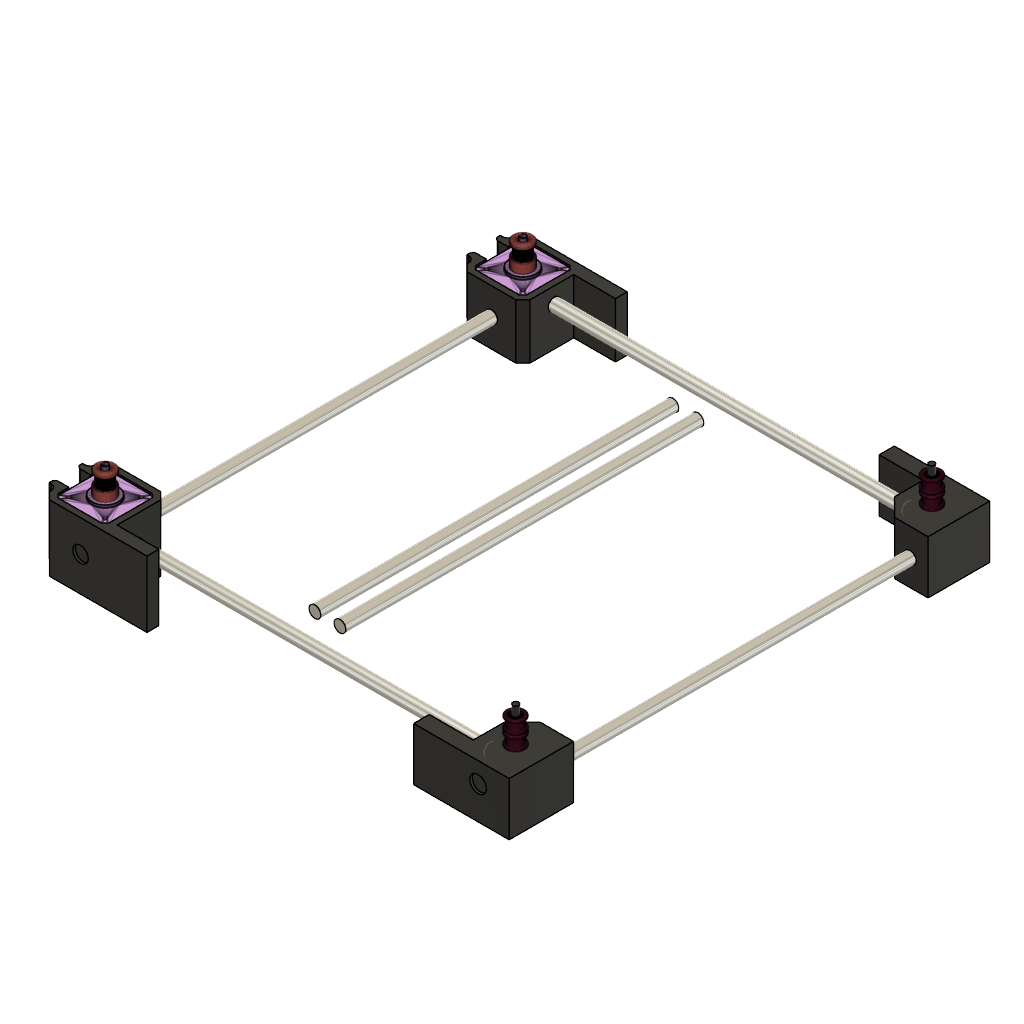
CoreXY  Assembly (Autodesk Fusion 360 archive; units mm, degrees)
design "Snakes And Ladders Player Final"
part number: 2026-09-22-01-13-54-061
Autodesk Fusion 360 part; units mm, degrees
other "Base Mesh Feature1"
other "Modify1"
sketch "Sketch1" plane through (0, 0, 0) normal (0, 1, 0) x (1, 0, 0)
  line L0 (21.3, -49.8) -> (-15.3, -49.8)
  line L1 (-15.3, -7.2) -> (21.3, -7.2)
  line L2 (24.3, -10.2) -> (24.3, -46.8)
  line L3 (-15.3, -49.8) -> (-18.3, -46.8)
  line L4 (21.3, -49.8) -> (24.3, -46.8)
  line L5 (21.3, -7.2) -> (24.3, -10.2)
  line L6 (-18.3, -10.2) -> (-15.3, -7.2)
  line L7 (-18.3, -37.5) -> (-25, -37.5)
  line L8 (-25, -37.5) -> (-25, -19.5)
  line L9 (-25, -19.5) -> (-18.3, -19.5)
  line L10 (-18.3, -46.8) -> (-18.3, -37.5)
  line L11 (-18.3, -19.5) -> (-18.3, -10.2)
  line L12 (-30, -14.5) -> (-23.3, -14.5)
  line L13 (-23.3, -14.5) -> (-23.3, -8.1289)
  line L14 (-23.3, -8.1289) -> (-17.3711, -2.2)
  line L15 (-17.3711, -2.2) -> (23.3711, -2.2)
  line L16 (23.3711, -2.2) -> (29.3, -8.1289)
  line L17 (29.3, -8.1289) -> (29.3, -48.8711)
  line L18 (23.3711, -54.8) -> (29.3, -48.8711)
  line L19 (23.3711, -54.8) -> (-17.3711, -54.8)
  line L20 (-17.3711, -54.8) -> (-23.3, -48.8711)
  line L21 (-23.3, -48.8711) -> (-23.3, -42.5)
  line L22 (-23.3, -42.5) -> (-30, -42.5)
  line L23 (-30, -42.5) -> (-30, -14.5)
  line L24 (-25, -37.5) -> (-30, -37.5)
  line L25 (-25, -19.5) -> (-30, -19.5)
  point P0 (24.3, -49.8)
  point P1 (-18.3, -49.8)
  point P2 (-18.3, -7.2)
  point P3 (24.3, -7.2)
  dimension "d1" = 42.6
  dimension "d2" = 42.6
  dimension "d3" = 3
  dimension "d4" = 3
  dimension "d5" = 3
  dimension "d6" = 3
  dimension "d7" = 3
  dimension "d8" = 3
  dimension "d9" = 3
  dimension "d10" = 3
  dimension "d11" = -5
  constraint horizontal L0
  constraint vertical L10
  constraint horizontal L1
  constraint vertical L2
  constraint coincident P1 L0
  constraint coincident P1 L10
  constraint coincident P0 L0
  constraint coincident P0 L2
  constraint coincident P3 L1
  constraint coincident P3 L2
  constraint coincident P2 L11
  constraint coincident P2 L1
  constraint horizontal L7
  constraint vertical L8
  constraint horizontal L9
  constraint collinear L10 L11
  constraint coincident L23 L24.end
  constraint perpendicular L23 L24
  constraint coincident L23 L25.end
  constraint perpendicular L23 L25
  measures "d1" distance of P0 P1
  measures "d2" distance of P0 P3
  measures "d3" distance of P1 L0.end
  measures "d4" distance of P1 L3.end
  measures "d5" distance of P0 L0.start
  measures "d6" distance of P0 L2.end
  measures "d7" distance of P3 L1.end
  measures "d8" distance of P3 L2.start
  measures "d9" distance of P2 L6.start
  measures "d10" distance of P2 L1.start
extrude "Extrude1" add sketch "Sketch1" along normal blind 35 contours L0 L1 L2 L3 L4 L5 L6 L7 L9 L10 L11 L12 L13 L14 L15 L16 L17 L18 L19 L20 L21 L22 L23 L24 L25 makes body 1
sketch "Sketch2" plane through (0, 0, 54.8) normal (0, 0, 1) x (1, 0, 0)
  line L0 (-17.3711, 0) -> (23.3711, 0)
  line L1 (23.3711, 0) -> (23.3711, 35)
  line L2 (23.3711, 35) -> (-17.3711, 35)
  line L3 (-17.3711, 35) -> (-17.3711, 0)
  circle A0 centre (3, 12) radius 5.075
  dimension "d14" = 10.15
  measures "d14" diameter of A0
extrude "Extrude2" cut sketch "Sketch2" against normal blind 2 contours A0 bodies 1
fillet "Fillet1" radius 5 2 edges at (-23.3, 17.5, 42.5) (-23.3, 17.5, 14.5) on bodies 1
fillet "Fillet2" radius 3 2 edges at (-30, 17.5, 19.5) (-30, 17.5, 37.5) on bodies 1
sketch "Sketch3" plane through (0, 0, 52.8) normal (0, 0, 1) x (1, 0, 0)
  circle A0 centre (3, 12) radius 5.075
  circle A1 centre (3, 12) radius 5
  dimension "d21" = 10
  constraint concentric A0 A1
  measures "d21" diameter of A1
extrude "Extrude3" add sketch "Sketch3" along normal blind 300 separate body contours A1 makes body 2
extrude "Extrude4" cut 1 faces at (27.6333, 0, 34.6) along direction (0, 1, 0) blind 1.4 on bodies 1 bodies 1
extrude "Extrude5" add sketch "Sketch1" against normal blind 3 separate body contours L0 L1 L2 L3 L4 L5 L6 L7 L8 L9 L10 L11 makes body 3
move_body "Move1" bodies 3 to x (1, 0, 0) y (0, 1, 0) z (0, 0, 1) at (0, 1.5, 0)
extrude "Extrude6" add 1 faces at (27.6333, 1.4, 34.6) along direction (0, -1, 0) blind 2.9 on bodies 1 bodies 1 3
extrude "Extrude7" add 1 faces at (-25, 0.5, 31.5) along direction (-1, 0, 0) blind 2 on bodies 1 bodies 1
copy_body "CopyPasteBodies1" bodies 1 makes body 4
move_body "Move2" bodies 4 to x (1, 0, 0) y (0, 1, 0) z (0, 0, 1) at (0, 0, 350)
extrude "Extrude8" add 1 faces at (4.3887, 10.3675, 402.8) along direction (0, 0, 1) blind 2 on bodies 4 bodies 4
sketch "Sketch4" plane through (0, 0, 352.2) normal (0, 0, -1) x (-1, 0, 0)
  line L0 (17.3711, -1.5) -> (17.3711, 35)
  line L1 (17.3711, 35) -> (-23.3711, 35)
  line L2 (-23.3711, 35) -> (-23.3711, -1.5)
  line L3 (-23.3711, -1.5) -> (17.3711, -1.5)
  circle A0 centre (-3, 12) radius 5.075
  dimension "d34" = 10.15
  measures "d34" diameter of A0
extrude "Extrude9" cut sketch "Sketch4" against normal blind 2 contours A0 bodies 4
other "CopyPasteMeshes1"
other "Modify2"
extrude "Extrude10" add 1 faces at (10.1, 1.5, 381.5) along direction (0, 1, 0) blind 9.5 on bodies 4 bodies 4
extrude "Extrude11" add 1 faces at (27.6333, 35, 372.4) along direction (0, 1, 0) blind 10 on bodies 4 bodies 4
extrude "Extrude12" cut 1 faces at (27.6333, 35, 34.6) along direction (0, -1, 0) blind 0.5 on bodies 1 bodies 1
extrude "Extrude13" cut 1 faces at (27.6333, 45, 372.4) along direction (0, -1, 0) blind 1 on bodies 4 bodies 4
sketch "Sketch5" plane through (29.3, 0, 0) normal (1, 0, 0) x (0, 0, -1)
  line L0 (-358.1289, 44) -> (-398.8711, 44)
  line L1 (-398.8711, 44) -> (-398.8711, -1.5)
  line L2 (-398.8711, -1.5) -> (-358.1289, -1.5)
  line L3 (-358.1289, -1.5) -> (-358.1289, 44)
  line L4 (-378.5, -1.5) -> (-378.5, 44)
  circle A0 centre (-378.5, 21.25) radius 5.075
  dimension "d45" = 10.15
  constraint midpoint L2 L4.start
  constraint midpoint L0 L4.end
  constraint midpoint L4 A0.centre
  measures "d45" diameter of A0
extrude "Extrude14" cut sketch "Sketch5" against normal blind 2 contours L4 A0 | L4 A0 bodies 4
move_face "MoveFace1" to x (0.707107, 0, -0.707107) y (0, 1, 0) z (0.707107, 0, 0.707107) at (-273.4627, 0, 137.5449) 1 faces at (25.3474, 13.6667, 402.8237) on bodies 4
move_face "MoveFace2" to x (0.707107, 0, -0.707107) y (0, 1, 0) z (0.707107, 0, 0.707107) at (5.2896, 0, 17.1702) 1 faces at (25.3474, 10.5, 4.1763) on bodies 1
sketch "Sketch6" plane through (29.3, 0, 0) normal (1, 0, 0) x (0, 0, -1)
  line L0 (-2.2, 34.5) -> (-48.8711, 34.5)
  line L1 (-48.8711, 34.5) -> (-48.8711, -1.5)
  line L2 (-48.8711, -1.5) -> (-2.2, -1.5)
  line L3 (-2.2, -1.5) -> (-2.2, 34.5)
  line L4 (-24.4315, 18.2164) -> (-24.4315, -1.5)
  circle A0 centre (-28.5, 21.25) radius 5.075
  dimension "d52" = 10.15
  constraint vertical L4
  constraint coincident L4.start A0
  measures "d52" diameter of A0
extrude "Extrude16" cut sketch "Sketch6" against normal blind 2 contours A0 bodies 1
sketch "Sketch8" plane through (29.3, 0, 0) normal (1, 0, 0) x (0, 0, -1)
  circle A0 centre (-378.5, 21.25) radius 5.075
  line L0 (-358.1289, 44) -> (-404.8, 44)
  line L1 (-404.8, 44) -> (-404.8, -1.5)
  line L2 (-404.8, -1.5) -> (-358.1289, -1.5)
  line L3 (-358.1289, -1.5) -> (-358.1289, 44)
  line L4 (-404.8, 44) -> (-394.8, 44)
  line L5 (-394.8, 44) -> (-394.8, -1.5)
  line L6 (-394.8, -1.5) -> (-404.8, -1.5)
  line L7 (-404.8, -1.5) -> (-404.8, 44)
  dimension "d55" = 10
  constraint horizontal L4
  constraint vertical L5
  constraint horizontal L6
  constraint vertical L7
  constraint coincident L0.end L1.start
  measures "d55" distance of L0.end L4.end
extrude "Extrude17" add sketch "Sketch8" along normal blind 35 contours L0 L1 L2 L4 L5 L6 L7 bodies 4
sketch "Sketch9" plane through (29.3, 0, 0) normal (1, 0, 0) x (0, 0, -1)
  circle A0 centre (-28.5, 21.25) radius 5.075
  line L0 (-2.2, 34.5) -> (-48.8711, 34.5)
  line L1 (-48.8711, 34.5) -> (-48.8711, -1.5)
  line L2 (-48.8711, -1.5) -> (-2.2, -1.5)
  line L3 (-2.2, -1.5) -> (-2.2, 34.5)
  line L4 (-2.2, 34.5) -> (-12.2, 34.5)
  line L5 (-12.2, 34.5) -> (-12.2, -1.5)
  line L6 (-12.2, -1.5) -> (-2.2, -1.5)
  line L7 (-2.2, -1.5) -> (-2.2, 34.5)
  dimension "d58" = 10
  constraint horizontal L4
  constraint vertical L5
  constraint horizontal L6
  constraint vertical L7
  constraint coincident L0.start L3.end
  measures "d58" distance of L0.start L4.end
extrude "Extrude18" add sketch "Sketch9" along normal blind 35 contours L0 L2 L3 L4 L5 L6 L7 bodies 1
sketch "Sketch11" plane through (27.3, 0, 0) normal (1, 0, 0) x (0, 0, -1)
  circle A0 centre (-28.5, 21.25) radius 5.075
  circle A1 centre (-28.5, 21.25) radius 5
  circle A2 centre (-378.5, 21.25) radius 5
  circle A3 centre (-378.5, 21.25) radius 5.075
  dimension "d61" = 10
  dimension "d62" = 10
  constraint concentric A0 A1
  constraint concentric A2 A3
  measures "d61" diameter of A1
  measures "d62" diameter of A2
extrude "Extrude19" add sketch "Sketch11" along normal blind 300 separate body contours A2 makes body 5
extrude "Extrude20" add sketch "Sketch6" along normal blind 300 separate body contours A0 makes body 6
sketch "Sketch12" plane through (0, 0, 0) normal (0, 1, 0) x (1, 0, 0)
  line L0 (328, -5) -> (368, -5)
  line L1 (368, -5) -> (368, -50)
  line L2 (368, -50) -> (328, -50)
  line L3 (328, -50) -> (328, -5)
  line L4 (328, -5) -> (293, -5)
  line L5 (293, -5) -> (293, -15)
  line L6 (293, -15) -> (328, -15)
  line L7 (328, -15) -> (328, -5)
  dimension "d69" = 35
  dimension "d70" = 10
  constraint horizontal L0
  constraint vertical L1
  constraint horizontal L2
  constraint vertical L3
  constraint horizontal L4
  constraint vertical L5
  constraint horizontal L6
  constraint vertical L7
  measures "d69" distance of L0.start L4.end
  measures "d70" distance of L0.start L6.end
extrude "Extrude22" add sketch "Sketch12" along normal blind 34.5 separate body makes body 7
sketch "Sketch13" plane through (328, 0, 0) normal (-1, 0, 0) x (0, 0, 1)
  line L0 (15, 0) -> (50, 0)
  line L1 (50, 0) -> (50, 34.5)
  line L2 (50, 34.5) -> (15, 34.5)
  line L3 (15, 34.5) -> (15, 0)
copy_body "CopyPasteBodies2" bodies 6 makes body 8
scale "Scale1" factor 1.015 about (329.3, 21.25, 33.575) bodies 8
combine "Combine1" operation cut target body 7 tool bodies 8
copy_body "CopyPasteBodies3" bodies 2 makes body 9
move_body "Move3" bodies 9 to x (1, 0, 0) y (0, 1, 0) z (0, 0, 1) at (350, 0, 0)
scale "Scale2" factor 1.015 about (348, 12, 352.8) bodies 9
combine "Combine2" operation cut target body 7 tool bodies 9
copy_body "CopyPasteBodies4" bodies 2 makes body 10
move_body "Move4" bodies 10 to x (1, 0, 0) y (0, 1, 0) z (0, 0, 1) at (350, 0, 0)
extrude "Extrude23" add 1 faces at (334.7418, 15.9986, 50) along direction (0, 0, 1) blind 4 on bodies 7 bodies 7
extrude "Extrude24" add 1 faces at (353.3868, 11.2137, 48.3) along direction (0, 0, 1) blind 4 on bodies 7 bodies 7
copy_body "CopyPasteBodies5" bodies 7 makes body 11
copy_body "CopyPasteBodies6" bodies 11 makes body 12
move_body "Move5" bodies 12 to x (1, 0, 0) y (0, 1, 0) z (0, 0, 1) at (0, 0, 400)
delete_body "RemoveBody1" bodies 12
delete_body "RemoveBody2" bodies 11
move_body "Move7" bodies 6 to x (1, 0, 0) y (0, 1, 0) z (0, 0, 1) at (-2, 0, 0)
extrude "Extrude25" add 1 faces at (293, 11.5, 8.3333) along direction (-1, 0, 0) blind 2 on bodies 7 bodies 7
extrude "Extrude26" add 1 faces at (328, 18.3274, 47.1725) along direction (-1, 0, 0) blind 3 on bodies 7 bodies 7
extrude "Extrude27" add 1 faces at (291, 11.5, 8.3333) along direction (-1, 0, 0) blind 3 on bodies 7 bodies 7
extrude "Extrude28" add 1 faces at (329.3, 22.0752, 32.1819) along direction (-1, 0, 0) blind 3 on bodies 7 bodies 7
copy_body "CopyPasteBodies7" bodies 7 makes body 13
move_body "Move8" bodies 13 to x (1, 0, 0) y (0, 1, 0) z (0, 0, 1) at (0, 0, 400)
mirror "Mirror2" about plane through (291, 0, 405) normal (0, 0, -1) of bodies 13 makes body 14
delete_body "RemoveBody3" bodies 13
move_body "Move9" bodies 14 to x (1, 0, 0) y (0, 1, 0) z (0, 0, 1) at (0, 0, -3)
extrude "Extrude29" add 1 faces at (332.7418, 15.9986, 353) along direction (0, 0, -1) blind 2 on bodies 14 bodies 14
chamfer "Chamfer3" distance 15 angle 45 1 edges at (325, 17.25, 54) on bodies 7
chamfer "Chamfer4" distance 15 angle 45 1 edges at (325, 17.25, 351) on bodies 14
sketch "Sketch14" plane through (0, 34.5, 0) normal (0, 1, 0) x (-1, 0, 0)
  line L0 (-340, 351) -> (-325, 366)
  line L1 (-325, 366) -> (-325, 392)
  line L2 (-325, 392) -> (-288, 392)
  line L3 (-288, 392) -> (-288, 402)
  line L4 (-288, 402) -> (-368, 402)
  line L5 (-368, 402) -> (-368, 351)
  line L6 (-368, 351) -> (-340, 351)
  line L7 (-325, 39) -> (-325, 15)
  line L8 (-368, 5) -> (-368, 54)
  line L9 (-325, 29) -> (-368, 29.5)
  line L10 (-368, 5) -> (-288, 5)
  line L11 (-346.5, 29.25) -> (-346.782, 5)
  line L12 (-368, 54) -> (-340, 54)
  line L13 (-346.5, 29.25) -> (-346.2122, 54)
  line L14 (-368, 376.5) -> (-325, 376.5)
  line L15 (-346.5, 376.5) -> (-346.5, 402)
  line L16 (-346.5, 376.5) -> (-346.5, 351)
  circle A0 centre (-346.5, 377.9623) radius 2.5
  circle A1 centre (-346.5, 29.25) radius 2.5
  dimension "d99" = 5
  dimension "d100" = 5
  constraint coincident L7 L9.start
  constraint midpoint L8 L9.end
  constraint midpoint L9 L11.start
  constraint coincident L10 L11.end
  constraint perpendicular L9 L11
  constraint coincident L12 L13.end
  constraint perpendicular L9 L13
  constraint midpoint L5 L14.start
  constraint coincident L1 L14.end
  constraint perpendicular L1 L14
  constraint midpoint L14 L15.start
  constraint coincident L4 L15.end
  constraint perpendicular L4 L15
  constraint coincident L6 L16.end
  constraint perpendicular L6 L16
  constraint coincident L15 A0.centre
  constraint coincident L11.start L13.start
  measures "d99" diameter of A0
  measures "d100" diameter of A1
extrude "Extrude30" add sketch "Sketch14" along normal blind 30 contours L14 L16 A0 | L14 L16 A0 | L14 L15 A0 | L14 L15 A0 | L9 L13 A1 | L9 L11 A1 | L9 L11 A1 | L9 L13 A1 bodies 7 14
other "Base Mesh Feature2"
other "CopyPasteMeshes2"
other "Modify3"
other "Modify4"
other "Base Mesh Feature3"
other "Scale1'"
other "Modify5"
other "Modify6"
other "CopyPasteMeshes3"
other "Modify7"
other "CopyPasteMeshes4"
other "Modify8"
copy_body "CopyPasteBodies8" bodies 10 makes body 15
move_body "Move10" bodies 15 to x (1, 0, 0) y (0, 1, 0) z (0, 0, 1) at (-170, 0, 0)
copy_body "CopyPasteBodies9" bodies 15 makes body 16
move_body "Move11" bodies 16 to x (1, 0, 0) y (0, 1, 0) z (0, 0, 1) at (0, 40, 0)
move_body "Move12" bodies 15 16 to x (1, 0, 0) y (0, 1, 0) z (0, 0, 1) at (0, -10, 0)
extrude "Extrude31" add 2 faces at (9.6397, -1.5, 369.5257) (9.6397, -1.5, 37.4743) along direction (0, -1, 0) blind 10 on bodies 1 4 bodies 4 1 2 6 7 10 14
extrude "Extrude32" add 2 faces at (358.6667, 0, 37.6667) (358.6667, 0, 368) along direction (0, -1, 0) blind 10 on bodies 7 14 bodies 7 14
move_body "Move13" bodies 10 14 6 16 4 15 1 7 5 2 to x (1, 0, 0) y (0, 1, 0) z (0, 0, 1) at (0, 12, 0)
other "Modify10"
move_face "MoveFace4" to x (1, 0, 0) y (0, 1, 0) z (0, 0, 1) at (0, 10, 0) 2 faces at (187.9938, 13.7508, 252.8) (187.9938, 53.7508, 252.8) on bodies 15 16
other "Modify11"
extrude "Extrude37" add 1 faces at (341.3333, 16.8333, 402) along direction (0, 0, 1) blind 3 on bodies 14 bodies 14
extrude "Extrude39" add 1 faces at (314.6667, 31.6667, 5) along direction (0, 0, -1) blind 2.8 on bodies 7 bodies 7
other "Modify12"
other "Modify13"
other "Modify14"
sketch "Sketch17" plane through (0, 0, 0) normal (0, 1, 0) x (1, 0, 0)
  line L0 (2.4676, -20.1372, 50) -> (347, -21, 50)
  spline S0 degree 5 poles (347, -21, 50) (347.2059, -21.0417, 50) (347.6215, -21.137, 50) (348.2562, -21.3153, 50) (349.1254, -21.6241, 50) (350.2424, -22.1293, 50) (351.3681, -22.7528, 50) (352.4534, -23.4907, 50) (353.4252, -24.3341, 50) (354.145, -25.267, 50) (354.6049, -26.2634, 50) (354.8671, -27.2941, 50) (354.9971, -28.3347, 50) (355.0372, -29.3687, 50) (354.8766, -30.4029, 50) (354.5609, -31.4357, 50) (354.229, -32.4579, 50) (354.0105, -33.4557, 50) (353.9724, -34.4143, 50) (353.9677, -35.3147, 50) (353.953, -36.1812, 50) (353.9466, -36.8814, 50) (353.9623, -37.4294, 50) (353.9853, -37.8076, 50) (354, -38, 50) knots 0 0 0 0 0 0 0.05 0.1 0.15 0.2 0.25 0.3 0.35 0.4 0.45 0.5 0.55 0.6 0.65 0.7 0.75 0.8 0.85 0.9 0.95 1 1 1 1 1 1
  line L1 (355.0079, -26.8451, 50) -> (354.9921, -31.1549, 50)
  line L2 (351.2331, -22.3821, 50) -> (354.7669, -25.6179, 50)
  line L3 (353.8189, -35.6231, 50) -> (354.1811, -40.3769, 50)
  line L4 (354.1386, -31.8186, 50) -> (353.8615, -36.1814, 50)
  line L5 (354, -38, 50) -> (354, -380, 50)
  spline S1 degree 5 poles (354, -380, 50) (353.9826, -380.3445, 50) (353.9264, -381.007, 50) (353.7775, -381.921, 50) (353.4496, -382.9796, 50) (352.8234, -384.034, 50) (351.9846, -384.8201, 50) (350.9451, -385.344, 50) (349.7289, -385.6215, 50) (348.3763, -385.6812, 50) (346.9496, -385.5699, 50) (345.5239, -385.3456, 50) (344.176, -385.0705, 50) (342.9743, -384.8034, 50) (341.9673, -384.5922, 50) (341.1742, -384.4674, 50) (340.5693, -384.4323, 50) (340.0834, -384.4625, 50) (339.6318, -384.5223, 50) (339.1357, -384.5758, 50) (338.5485, -384.6015, 50) (337.9886, -384.5918, 50) (337.5151, -384.5661, 50) (337.1756, -384.5408, 50) (337, -384.5261, 50) knots 0 0 0 0 0 0 0.05 0.1 0.15 0.2 0.25 0.3 0.35 0.4 0.45 0.5 0.55 0.6 0.65 0.7 0.75 0.8 0.85 0.9 0.95 1 1 1 1 1 1
  line L6 (337, -384.5261, 50) -> (183.3789, -384.5261, 50)
  point P0 (353, -24)
  point P1 (355, -29)
  point P2 (354, -34)
  point P3 (349.5273, -385.5878)
  point P4 (341.4985, -384.5261)
  point P5 (339.5742, -384.5261)
move_face "MoveFace5" to x (1, 0, 0) y (0, 1, 0) z (0, 0, 1) at (-30, -40, 0) 1 faces at (187.9938, 63.7508, 252.8) on bodies 16
move_face "MoveFace6" to x (1, 0, 0) y (0, 1, 0) z (0, 0, 1) at (0, 10, 0) 2 faces at (187.9938, 23.7508, 252.8) (157.9938, 23.7508, 252.8) on bodies 15 16
sketch "Sketch19" plane through (0, 0, 404.8) normal (0, 0, 1) x (1, 0, 0)
  line L0 (64.3, 56) -> (-17.3711, 56)
  line L1 (-17.3711, 56) -> (-17.3711, 0.5)
  line L2 (-17.3711, 0.5) -> (64.3, 0.5)
  line L3 (64.3, 0.5) -> (64.3, 56)
  circle A0 centre (8.6289, 29.5) radius 6.5
  dimension "d151" = 13
  measures "d151" diameter of A0
sketch "Sketch20" plane through (0, 0, 2.2) normal (0, 0, -1) x (-1, 0, 0)
  line L0 (17.3711, 46.5) -> (-64.3, 46.5)
  line L1 (-64.3, 46.5) -> (-64.3, 0.5)
  line L2 (-64.3, 0.5) -> (17.3711, 0.5)
  line L3 (17.3711, 0.5) -> (17.3711, 46.5)
  circle A0 centre (-8.6289, 29.5) radius 6.5
  dimension "d148" = 13
  measures "d148" diameter of A0
sketch "Sketch23" plane through (0, 0, 405) normal (0, 0, 1) x (1, 0, 0)
  line L0 (368, 2) -> (368, 46.5)
  line L1 (368, 46.5) -> (288, 46.5)
  line L2 (288, 46.5) -> (288, 2)
  line L3 (288, 2) -> (368, 2)
  line L4 (368, 46.5) -> (342, 46.5)
  line L5 (342, 46.5) -> (342, 29.5)
  line L6 (342, 29.5) -> (368, 29.5)
  line L7 (368, 29.5) -> (368, 46.5)
  circle A0 centre (342, 29.5) radius 7
  dimension "d135" = 26
  dimension "d136" = 17
  dimension "d137" = 14
  constraint horizontal L4
  constraint vertical L5
  constraint horizontal L6
  constraint vertical L7
  constraint coincident L0.end L1.start
  constraint coincident L5.end L6.start
  measures "d135" distance of L0.end L4.end
  measures "d136" distance of L0.end L6.end
  measures "d137" diameter of A0
extrude "Extrude42" cut sketch "Sketch23" against normal blind 2.2 contours L5 L6 A0 | L5 L6 A0 bodies 14
sketch "Sketch24" plane through (0, 0, 2.2) normal (0, 0, -1) x (-1, 0, 0)
  line L0 (-288, 2) -> (-288, 46.5)
  line L1 (-288, 46.5) -> (-368, 46.5)
  line L2 (-368, 46.5) -> (-368, 2)
  line L3 (-368, 2) -> (-288, 2)
  line L4 (-368, 46.5) -> (-342, 46.5)
  line L5 (-342, 46.5) -> (-342, 29.5)
  line L6 (-342, 29.5) -> (-368, 29.5)
  line L7 (-368, 29.5) -> (-368, 46.5)
  circle A0 centre (-342, 29.5) radius 7
  dimension "d140" = 26
  dimension "d141" = 17
  dimension "d142" = 14
  constraint horizontal L4
  constraint vertical L5
  constraint horizontal L6
  constraint vertical L7
  constraint coincident L1.end L2.start
  constraint coincident L5.end L6.start
  measures "d140" distance of L1.end L4.end
  measures "d141" distance of L1.end L6.end
  measures "d142" diameter of A0
extrude "Extrude43" cut sketch "Sketch24" against normal blind 2.2 contours L5 L6 A0 | L5 L6 A0 bodies 7
extrude "Extrude44" cut sketch "Sketch19" against normal blind 2.2 contours A0 bodies 4
extrude "Extrude45" cut sketch "Sketch20" against normal blind 2.2 contours A0 bodies 1
sketch "Sketch25" plane through (0, 0, 0) normal (0, 1, 0) x (1, 0, 0)
sketch "Sketch26" plane through (0, 0, 404.8) normal (0, 0, 1) x (1, 0, 0)
  circle A0 centre (8.6289, 29.5) radius 6.5
  line L0 (64.3, 56) -> (-17.3711, 56)
  line L1 (-17.3711, 56) -> (-17.3711, 0.5)
  line L2 (-17.3711, 0.5) -> (64.3, 0.5)
  line L3 (64.3, 0.5) -> (64.3, 56)
  line L4 (8.6289, 29.5) -> (-30, 29.5)
  line L5 (-30, 29.5) -> (-30, 0.5)
  line L6 (-30, 0.5) -> (8.6289, 0.5)
  line L7 (8.6289, 0.5) -> (8.6289, 29.5)
  constraint horizontal L4
  constraint vertical L5
  constraint horizontal L6
  constraint vertical L7
  constraint coincident A0.centre L4.start
move_body "Move15" bodies 15 to x (1, 0, 0) y (0, 1, 0) z (0, 0, 1) at (-9, 0, 0)
equation "d4 = d3"
equation "d6 = d5"
equation "d8 = d7"
equation "d10 = d9"
named bodies: "Motor Housing Left", "Structural Rod 1", "Motor Housing", "Motor Housing Right", "Main Rail Left", "Main Rail Right", "Top Left Bracket", "Structural Rod 1 (1)", "Structural Rod 2", "Top Left Bracket (1)", "Top Left Bracket (1) (1)", "Top Left Bracket (2)", "Top Right Bracket", "Main Gondola Rod 1", "Main Gondola Rod 2"
